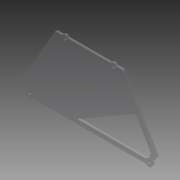
# Autodesk Inventor part: Top Plat
Saved by Autodesk Inventor 2015 (Build 190159000, 159)
## iProperties
Created: 2016-10-14
Part Number: Top Plat
Material: Generic
Document SubType Name: Modeling
Designer: James Yelland
Density: 1 g/cm^3
Appearance: Default
Author: James Yelland
Autodesk Inventor part; units mm, degrees
ref_plane "YZ Plane" through (0, 0, 0) normal (1, 0, 0) x (0, 1, 0)
ref_plane "XZ Plane" through (0, 0, 0) normal (0, 1, 0) x (-1, 0, 0)
ref_plane "XY Plane" through (0, 0, 0) normal (0, 0, 1) x (1, 0, 0)
sketch "Sketch1" plane through (0, 0, 0) normal (0, 1, 0) x (-1, 0, 0)
  circle A0 centre (32.6132, 75.9327) radius 1.6
  circle A1 centre (-32.6132, 75.9327) radius 1.6
  circle A2 centre (80.7596, -11.9856) radius 1.6
  circle A3 centre (-80.7596, -11.9856) radius 1.6
  circle A4 centre (80.7596, -11.9856) radius 5
  circle A5 centre (32.6132, 75.9327) radius 5
  circle A6 centre (-32.6132, 75.9327) radius 5
  circle A7 centre (-80.7596, -11.9856) radius 5
  line L0 (-90.2776, 1.5) -> (-46.4378, 77.4327)
  line L1 (46.4378, 77.4327) -> (90.2776, 1.5)
  line L2 (-83.3494, 1.5) -> (-42.9737, 71.4327)
  line L3 (36.6132, 72.9327) -> (40.3756, 72.9327)
  line L4 (42.9737, 71.4327) -> (83.3494, 1.5)
  line L5 (83.3494, -1.5) -> (80.1615, -7.0215)
  line L6 (85.3577, -10.0215) -> (90.2776, -1.5)
  line L7 (43.8397, 78.9327) -> (36.6132, 78.9327)
  line L8 (28.6132, 72.9327) -> (-28.6132, 72.9327)
  line L9 (-28.6132, 78.9327) -> (28.6132, 78.9327)
  line L10 (-36.6132, 72.9327) -> (-40.3756, 72.9327)
  line L11 (-36.6132, 78.9327) -> (-43.8397, 78.9327)
  line L12 (-83.3494, -1.5) -> (-80.1615, -7.0215)
  line L13 (-85.3577, -10.0215) -> (-90.2776, -1.5)
  line L14 (-80.7596, -11.9856) -> (-77.7596, -11.9856) construction
  line L15 (76.7596, -14.9856) -> (-76.7596, -14.9856)
  line L16 (-76.7596, -8.9856) -> (76.7596, -8.9856)
  arc A8 (90.2776, -1.5) -> (90.2776, 1.5) centre (87.6795, 0) ccw
  arc A9 (83.3494, -1.5) -> (83.3494, 1.5) centre (80.7513, 0) ccw
  arc A10 (46.4378, 77.4327) -> (43.8397, 78.9327) centre (43.8397, 75.9327) ccw
  arc A11 (42.9737, 71.4327) -> (40.3756, 72.9327) centre (40.3756, 69.9327) ccw
  arc A12 (-43.8397, 78.9327) -> (-46.4378, 77.4327) centre (-43.8397, 75.9327) ccw
  arc A13 (-40.3756, 72.9327) -> (-42.9737, 71.4327) centre (-40.3756, 69.9327) ccw
  arc A14 (-83.3494, 1.5) -> (-83.3494, -1.5) centre (-80.7513, 0) ccw
  arc A15 (-90.2776, 1.5) -> (-90.2776, -1.5) centre (-87.6795, 0) ccw
  line L17 (42.9737, 71.4327) -> (45.4737, 67.1025)
  line L18 (45.4737, 67.1025) -> (48.4737, 61.9064)
  line L19 (-42.9737, 71.4327) -> (-45.4737, 67.1025)
  line L20 (-45.4737, 67.1025) -> (-48.4737, 61.9064)
  line L21 (-63.1615, 36.4663) -> (15.5635, -8.9856)
  line L22 (-63.1615, 36.4663) -> (27.7423, 36.4663) construction
  point P0 (0, 0)
  point P1 (0, 0)
  point P2 (45.5718, 78.9327)
  point P3 (91.1436, 0)
  point P4 (0, 0)
  point P5 (-84.2154, 0)
  point P6 (-42.1077, 72.9327)
  point P7 (-80.8494, -5.8301)
  point P8 (-74.3148, -8.9856)
  point P9 (80.8494, -5.8301)
  point P10 (74.3148, -8.9856)
  dimension "d0" = 3.2
  dimension "d1" = 3.2
  dimension "d2" = 3.2
  dimension "d3" = 10
  dimension "d4" = 10
  dimension "d24" = 3
  dimension "d27" = 5
  dimension "d29" = 6
  dimension "d31" = 5
  dimension "d33" = 6
  dimension "d35" = 30
  constraints: 46 end point, 32 point on circle, 17 point on line, 16 centre point, 16 tangent, 7 equal radius, 6 coincident, 3 horizontal, 1 equal length, 1 midpoint, 1 parallel, 4 other
  measures "d0" diameter of A0
  measures "d1" diameter of A2
  measures "d2" diameter of A3
  measures "d3" diameter of A4
  measures "d4" diameter of A5
  measures "d24" radius of A8
  measures "d27" distance of L4.start L17.end
  measures "d29" distance of L17.end L18.end
  measures "d31" distance of L2.end L19.end
  measures "d33" distance of L19.end L20.end
  measures "d35" angle of L21 L22
extrude "Extrusion1" add sketch "Sketch1" along normal blind 3 contours A4 | A4 L5 A9 L4 A11 L3 A5 L7 A10 L1 A8 L6 | L15 A7 L16 A4 | A4 L16 L21 L2 A13 L10 A6 L8 A5 L3 A11 L4 A9 L5 | A7 | L13 A15 L0 A12 L11 A6 L10 A13 L2 A14 L12 A7 | A5 | A5 L8 A6 L9 | A6
body "Solid1"
